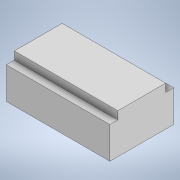
# Autodesk Inventor part: sensorMount
Saved by Autodesk Inventor 2021 (Build 250183000, 183)
## iProperties
Created: 2021-01-13
Part Number: sensorMount
Material: Generic
Document SubType Name: Modeling
Designer: awitc
Density: 1 g/cm^3
Appearance: Default
Author: awitc
Autodesk Inventor part; units mm, degrees
ref_plane "YZ Plane" through (0, 0, 0) normal (1, 0, 0) x (0, 1, 0)
ref_plane "XZ Plane" through (0, 0, 0) normal (0, 1, 0) x (-1, 0, 0)
ref_plane "XY Plane" through (0, 0, 0) normal (0, 0, 1) x (1, 0, 0)
sketch "Sketch1" plane through (0, 0, 0) normal (0, 1, 0) x (-1, 0, 0)
  line L0 (0, 4) -> (-20, 4)
  line L1 (-20, 4) -> (-20, -4)
  line L2 (-20, -4) -> (0, -4)
  circle A0 centre (-20, 0) radius 4
  circle A1 centre (-20, 0) radius 2.5
  line L3 (-20, -4) -> (-30, -4)
  line L4 (-30, -4) -> (-30, 4)
  line L5 (-30, 4) -> (-20, 4)
  line L6 (-20, 4) -> (-20, -4)
  circle A2 centre (4, 0) radius 4
  circle A3 centre (4, 0) radius 2.5
  line L7 (0, 4) -> (4, 4)
  line L8 (4, -4) -> (0, -4)
  line L9 (0, 0) -> (-1.5, 0)
  line L10 (-1.5, 0) -> (-14.5, 0)
  line L11 (-14.5, 0) -> (-14.5, -4)
  line L12 (-1.5, 0) -> (-1.5, -4)
  line L13 (-1.5, 0) -> (-1.5, 4)
  line L14 (-14.5, 0) -> (-14.5, 4)
  dimension "d0" = 20
  dimension "d1" = 5
  dimension "d2" = 10
  dimension "d3" = 5
  dimension "d4" = 1.5
  dimension "d5" = 13
  constraints: 30 end point, 7 point on line, 4 parallel, 4 perpendicular, 3 centre point, 3 horizontal, 2 coincident, 2 point on circle, 2 tangent, 1 midpoint, 1 vertical alignment, 2 other
  measures "d0" distance of L2.end L1.end
  measures "d1" diameter of A1
  measures "d2" distance of L4.end L5.end
  measures "d3" diameter of A3
  measures "d4" distance of L9.start L9.end
  measures "d5" distance of L9.end L10.end
extrude "Extrusion1" add sketch "Sketch1" along normal blind 5 contours L13 L10 L14 L0 | L12 L2 L11 L10
sketch "Sketch2" plane through (0, 5, 0) normal (0, 1, 0) x (1, 0, 0)
  line L0 (14.5, 4) -> (1.5, 4) projected
  line L1 (1.5, 4) -> (1.5, 3)
  line L2 (1.5, 4) -> (1.5, -4) projected
  line L3 (1.5, 3) -> (1.5, -3)
  line L4 (1.5, 3) -> (14.5, 3)
  line L5 (14.5, 3) -> (14.5, -3)
  line L6 (14.5, -4) -> (14.5, 4) projected
  line L7 (1.5, -3) -> (14.5, -3)
  line L8 (1.5, -4) -> (14.5, -4) projected
  line L9 (14.5, -4) -> (1.5, -4)
  point P0 (0, 0)
  dimension "d8" = 1
  dimension "d9" = 6
  constraints: 12 end point, 3 point on line, 2 horizontal, 1 perpendicular
  measures "d8" distance of L0.end L1.end
  measures "d9" distance of L1.end L3.end
extrude "Extrusion2" cut sketch "Sketch2" against normal blind 1 contours L6 L4 L1 L0 | L6 L8 L2 L7
body "Solid1"
